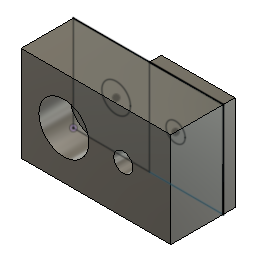
LRF Support Bracket v3 (Autodesk Fusion 360 design; units mm, degrees)
Autodesk Fusion 360 part; units mm, degrees
sketch "Sketch1" plane through (0, 0, 0) normal (0, 0, 1) x (1, 0, 0)
  line L0 (0, 0) -> (16.002, 0)
  line L1 (16.002, 0) -> (16.002, 10.16)
  line L2 (16.002, 10.16) -> (0, 10.16)
  line L3 (0, 10.16) -> (0, 0)
  circle A0 centre (10.922, 5.08) radius 1.016
  circle A1 centre (4.572, 5.08) radius 1.524
  line L4 (16.002, 10.16) -> (8.128, 10.16)
  line L5 (8.128, 10.16) -> (8.128, 0)
  line L6 (8.128, 0) -> (16.002, 0)
  line L7 (16.002, 0) -> (16.002, 10.16)
  dimension "d1" = 16.002
  dimension "d2" = 10.16
  dimension "d3" = 2.032
  dimension "d4" = 3.048
  dimension "d5" = 5.08
  dimension "d6" = 5.08
  dimension "d7" = 4.572
  dimension "d8" = 6.35
  dimension "d21" = 7.874
  constraint horizontal L0
  constraint vertical L1
  constraint horizontal L2
  constraint vertical L3
  constraint coincident L0.start L3.end
  constraint horizontal L4
  constraint vertical L5
  constraint horizontal L6
  constraint vertical L7
  measures "d1" distance of L0.start L0.end
  measures "d2" distance of L0.start L2.end
  measures "d3" diameter of A0
  measures "d4" diameter of A1
  measures "d5" distance of L2 A1.centre
  measures "d6" distance of L2 A0.centre
  measures "d7" distance of L3 A1.centre
  measures "d8" distance of A0.centre A1.centre
  measures "d21" distance of L1.end L4.end
extrude "Extrude6" add sketch "Sketch1" against normal blind 1.27 contours L0 L1 L2 L4 L5 L6 L7 makes body 1
extrude "Extrude1" add sketch "Sketch1" along normal blind 5.588 separate body makes body 2
extrude "Extrude2" add sketch "Sketch1" along normal blind 5.588 contours A0 bodies 2
extrude "Extrude3" cut sketch "Sketch1" along normal blind 5.588 contours A0 bodies 2
sketch "Sketch2" plane through (0, 0, 5.588) normal (0, 0, 1) x (1, 0, 0)
  circle A0 centre (4.572, 5.08) radius 1.524
  line L0 (0, 10.16) -> (0, 0)
  line L1 (0, 0) -> (16.002, 0)
  line L2 (16.002, 0) -> (16.002, 10.16)
  line L3 (16.002, 10.16) -> (0, 10.16)
  circle A1 centre (4.572, 5.08) radius 2.667
  line L4 (0, 10.16) -> (8.89, 10.16)
  line L5 (8.89, 10.16) -> (8.89, 0)
  line L6 (8.89, 0) -> (0, 0)
  line L7 (0, 0) -> (0, 10.16)
  circle A2 centre (10.922, 5.08) radius 1.016
  dimension "d15" = 5.334
  dimension "d18" = 8.89
  constraint concentric A0 A1
  constraint horizontal L4
  constraint vertical L5
  constraint horizontal L6
  constraint vertical L7
  constraint coincident L0.start L3.end
  measures "d15" diameter of A1
  measures "d18" distance of L0.start L4.end
extrude "Extrude4" cut sketch "Sketch2" against normal blind 3.302 contours A1 bodies 2
